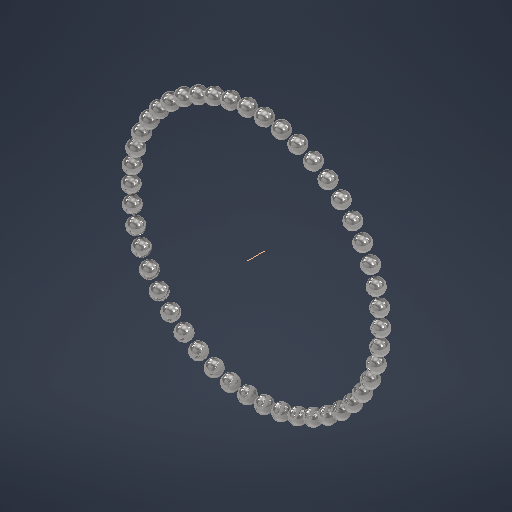
# Autodesk Inventor part: Plataforma_giratória_esfera
Saved by Autodesk Inventor 2025.2 (Build 292293000, 293)
## iProperties
Created: 2025-05-29
Part Number: Plataforma_giratória_esfera
Material: Generic
Document SubType Name: Modeling
Designer: Tiago
Density: 1 g/cm^3
Appearance: Generic
Author: Tiago
Autodesk Inventor part; units mm, degrees
ref_plane "YZ Plane" through (0, 0, 0) normal (1, 0, 0) x (0, 1, 0)
ref_plane "XZ Plane" through (0, 0, 0) normal (0, 1, 0) x (-1, 0, 0)
ref_plane "XY Plane" through (0, 0, 0) normal (0, 0, 1) x (1, 0, 0)
sketch "Sketch2" plane through (0, 0, 0) normal (0, 0, 1) x (1, 0, 0)
  circle A0 centre (0, 0) radius 32.9175
  circle A1 centre (-32.9175, 0) radius 2
  line L0 (-34.9175, 0) -> (-30.9175, 0)
  dimension "d3" = 65.835
  dimension "d4" = 4
  constraints: 2 end point, 2 point on circle, 1 centre point, 1 coincident, 1 horizontal, 1 horizontal alignment, 2 other
  measures "d4" diameter of A1
revolve "Revolution2" add sketch "Sketch2" angle 360 about axis through (-34.9175, 0, 0) along (1, 0, 0) picked at (-32.2647, 0.3678) picked at (-33.5134, 0.5167) contours A1 L0 A0 | A0 L0 A1
pattern_circular "Circular Pattern1" count 46 over 360 about axis through (0, 0, -10) along (0, 0, 1) of "Revolution2"
body "Solid2"
